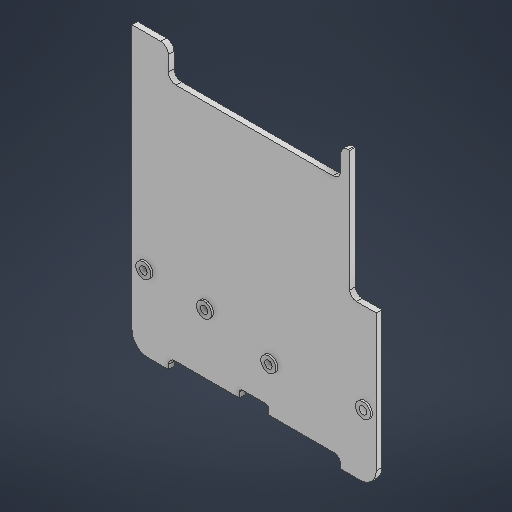
# Autodesk Inventor part: 第二层板
Saved by Autodesk Inventor 2025 (Build 290162000, 162)
## iProperties
Created: 2025-11-17
Part Number: 第二层板
Material: 常规
Document SubType Name: Modeling
Designer: XH
Density: 1 g/cm^3
Appearance: 默认
Author: XH
Autodesk Inventor part; units mm, degrees
ref_plane "YZ Plane" through (0, 0, 0) normal (1, 0, 0) x (0, 1, 0)
ref_plane "XZ Plane" through (0, 0, 0) normal (0, 1, 0) x (-1, 0, 0)
ref_plane "XY Plane" through (0, 0, 0) normal (0, 0, 1) x (1, 0, 0)
sketch "草图1" plane through (0, 0, 0) normal (0, 0, 1) x (1, 0, 0)
  arc A0 (28.0311, -36.5071) -> (33.0311, -31.5071) centre (28.0311, -31.5071) ccw
  line L0 (33.0311, -31.5071) -> (33.0311, 38.9929)
  line L1 (-32.9689, 38.9929) -> (-32.9689, -31.5071)
  arc A1 (-32.9689, -31.5071) -> (-27.9689, -36.5071) centre (-27.9689, -31.5071) ccw
  line L2 (3.8993, -36.5071) -> (3.8993, -31.5071)
  line L3 (3.8993, -36.5071) -> (28.0311, -36.5071)
  line L4 (-27.9689, -36.5071) -> (-3.837, -36.5071)
  line L5 (-3.837, -31.5071) -> (-3.837, -36.5071)
  spline S0 degree 3 poles (-2.9689, -30.724) (-3.0651, -30.724) (-3.1616, -30.7385) (-3.4015, -30.8136) (-3.5389, -30.8982) (-3.7629, -31.1465) (-3.837, -31.3265) (-3.837, -31.5071) knots 0 0 0 0 0.223691 0.223691 0.581598 0.581598 1 1 1 1
  line L6 (3.0311, -30.724) -> (-2.9689, -30.724)
  spline S1 degree 3 poles (3.8993, -31.5071) (3.8993, -31.3255) (3.8262, -31.1474) (3.5998, -30.8969) (3.4634, -30.8135) (3.224, -30.7385) (3.1274, -30.724) (3.0311, -30.724) knots 0 0 0 0 0.418614 0.418614 0.77639 0.77639 1 1 1 1
  line L7 (33.0311, 38.9929) -> (-32.9689, 38.9929)
  point P0 (22.1238, -37.5165)
extrude "拉伸1" add sketch "草图1" along normal blind 1.5
sketch "草图2" plane through (0, 0, 1.5) normal (0, 0, 1) x (1, 0, 0)
  line L0 (-21.8762, -36.6656) -> (22.1238, -36.6656)
  line L1 (22.1238, -36.6656) -> (-21.8762, -36.6656)
  line L2 (-21.8762, -36.6656) -> (-21.8762, -33.6656)
  line L3 (-21.8762, -33.6656) -> (22.1238, -33.6656)
  line L4 (22.1238, -33.6656) -> (22.1238, -36.6656)
  line L5 (-27.7974, -36.6656) -> (28.2026, -36.6656) projected
  point P0 (0, 0)
  point P1 (-21.8762, -36.6656)
  dimension "d3" = 3
  constraints: 10 end point, 2 parallel, 1 collinear, 1 horizontal, 1 perpendicular
  measures "d3" distance of L1.end L2.end
extrude "拉伸2" cut sketch "草图2" against normal blind 2
fillet "圆角1" radius 1 2 edges at (-21.8762, -33.6656, 0.75) (22.1238, -33.6656, 0.75)
sketch "草图3" plane through (0, 0, 1.5) normal (0, 0, 1) x (1, 0, 0)
  line L0 (26.0311, 37.3344) -> (33.1347, 37.3344)
  line L1 (33.0311, 37.4521) -> (33.0311, 5.3344)
  line L2 (33.0311, 5.3344) -> (26.0311, 5.3344)
  line L3 (26.0311, 5.3344) -> (26.0311, 37.3344)
  line L4 (33.0311, -31.5071) -> (33.0311, 38.9929) projected
  line L5 (33.2026, 37.3344) -> (-32.7974, 37.3344) projected
  point P0 (0, 0)
  point P1 (33.2026, -31.6656)
  point P2 (33.0311, 37.3344)
  point P3 (33.0311, 38.9929)
  dimension "d10" = 7
  dimension "d11" = 32
  constraints: 8 end point, 1 collinear, 1 horizontal, 1 parallel, 1 perpendicular, 1 vertical, 1 other
  measures "d10" distance between parallel lines of L1 L3
  measures "d11" distance between parallel lines of L0 L2
extrude "拉伸3" cut sketch "草图3" against normal blind 10
fillet "圆角2" radius 1 1 edges at (26.0311, 5.3344, 0.75)
sketch "草图4" plane through (0, 0, 1.5) normal (0, 0, 1) x (1, 0, 0)
  line L0 (33.0311, 5.3344) -> (27.0311, 5.3344) projected
  arc A0 (26.0311, 6.3344) -> (27.0311, 5.3344) centre (27.0311, 6.3344) ccw projected
  line L1 (26.0311, 6.3344) -> (26.0311, 37.3344) projected
  line L2 (-32.9689, 38.9929) -> (-32.9689, -31.5071) projected
  arc A1 (-32.9689, -31.5071) -> (-27.9689, -36.5071) centre (-27.9689, -31.5071) ccw projected
  line L3 (-21.8762, -36.5071) -> (-21.8762, -34.6656) projected
  arc A2 (-20.8762, -33.6656) -> (-21.8762, -34.6656) centre (-20.8762, -34.6656) ccw projected
  line L4 (-20.8762, -33.6656) -> (-3.837, -33.6656) projected
  arc A3 (22.1238, -34.6656) -> (21.1238, -33.6656) centre (21.1238, -34.6656) ccw projected
  line L5 (22.1238, -34.6656) -> (22.1238, -36.5071) projected
  arc A4 (28.0311, -36.5071) -> (33.0311, -31.5071) centre (28.0311, -31.5071) ccw projected
  line L6 (33.0311, -31.5071) -> (33.0311, 5.3344) projected
  line L7 (-32.2293, 38.2533) -> (25.2916, 38.2533)
  line L8 (25.2916, 38.2533) -> (25.2916, 6.3344)
  arc A5 (25.2916, 6.3344) -> (27.0311, 4.5949) centre (27.0311, 6.3344) ccw
  line L9 (27.0311, 4.5949) -> (32.2916, 4.5949)
  line L10 (32.2916, 4.5949) -> (32.2916, -31.5071)
  arc A6 (28.0311, -35.7676) -> (32.2916, -31.5071) centre (28.0311, -31.5071) ccw
  line L11 (28.0311, -35.7676) -> (22.8633, -35.7676)
  line L12 (22.8633, -35.7676) -> (22.8633, -34.6656)
  arc A7 (22.8633, -34.6656) -> (21.1238, -32.926) centre (21.1238, -34.6656) ccw
  line L13 (21.1238, -32.926) -> (-20.8762, -32.926)
  arc A8 (-20.8762, -32.926) -> (-22.6158, -34.6656) centre (-20.8762, -34.6656) ccw
  line L14 (-22.6158, -34.6656) -> (-22.6158, -35.7676)
  line L15 (-22.6158, -35.7676) -> (-27.9689, -35.7676)
  arc A9 (-32.2293, -31.5071) -> (-27.9689, -35.7676) centre (-27.9689, -31.5071) ccw
  line L16 (-32.2293, -31.5071) -> (-32.2293, 38.2533)
  line L17 (26.0311, 37.3344) -> (33.0311, 37.3344) projected
  line L18 (33.0311, 37.3344) -> (33.0311, 38.9929) projected
  line L19 (33.0311, 38.9929) -> (-32.9689, 38.9929) projected
  line L20 (-27.9689, -36.5071) -> (-21.8762, -36.5071) projected
  line L21 (-3.837, -33.6656) -> (-3.837, -31.5071) projected
  spline S0 degree 3 poles (-3.837, -31.5071) (-3.837, -31.3265) (-3.7629, -31.1465) (-3.5389, -30.8982) (-3.4015, -30.8136) (-3.1616, -30.7385) (-3.0651, -30.724) (-2.9689, -30.724) knots 0 0 0 0 0.418402 0.418402 0.776309 0.776309 1 1 1 1 projected
  line L22 (-2.9689, -30.724) -> (3.0311, -30.724) projected
  spline S1 degree 3 poles (3.0311, -30.724) (3.1274, -30.724) (3.224, -30.7385) (3.4634, -30.8135) (3.5998, -30.8969) (3.8262, -31.1474) (3.8993, -31.3255) (3.8993, -31.5071) knots 0 0 0 0 0.22361 0.22361 0.581386 0.581386 1 1 1 1 projected
  line L23 (3.8993, -31.5071) -> (3.8993, -33.6656) projected
  line L24 (3.8993, -33.6656) -> (21.1238, -33.6656) projected
  line L25 (22.1238, -36.5071) -> (28.0311, -36.5071) projected
  point P0 (0, 0)
  constraints: 20 end point, 10 point on circle, 5 centre point, 11 other
extrude "拉伸4" cut sketch "草图4" against normal blind 10 contours L6 A4 L25 L5 A3 L24 L23 L13 A7 L12 L11 A6 L10 L9 A5 L8 L7 L16 A9 L15 L14 A8 L21 L4 A2 L3 L20 A1 L2 L19 L18 L17 L1 A0 L0
sketch "草图5" plane through (0, 0, 1.5) normal (0, 0, 1) x (1, 0, 0)
  line L0 (25.2916, 38.2533) -> (-32.2293, 38.2533) projected
  line L1 (-22.6158, -35.7676) -> (22.8633, -35.7676)
  line L2 (22.8633, -35.7676) -> (22.8633, 38.2533)
  line L3 (22.8633, 38.2533) -> (-22.6158, 38.2533)
  line L4 (-22.6158, 38.2533) -> (-22.6158, -35.7676)
  line L5 (22.8633, -34.6656) -> (22.8633, -35.7676) projected
  line L6 (-22.6158, -35.7676) -> (-22.6158, -34.6656) projected
  line L7 (-27.9689, -35.7676) -> (-22.6158, -35.7676) projected
  line L8 (-22.6158, 30.2533) -> (22.8633, 30.2533)
  point P0 (0, 0)
  point P1 (-22.6158, 38.2533)
  dimension "d16" = 8
  constraints: 10 end point, 3 collinear, 3 point on line, 2 parallel, 2 perpendicular, 1 horizontal
  measures "d16" distance between parallel lines of L3 L8
extrude "拉伸5" cut sketch "草图5" against normal blind 10 contours L2 L8 L4 L0
fillet "圆角3" radius 2 4 edges at (22.8633, 38.2533, 0.75) (22.8633, 30.2533, 0.75) (-22.6158, 38.2533, 0.75) (-22.6158, 30.2533, 0.75)
sketch "草图6" plane through (0, 0, 1.5) normal (0, 0, 1) x (1, 0, 0)
  line L0 (29.89, -22.1052) -> (29.89, -32.1052) projected
  line L1 (29.89, -32.1052) -> (18.89, -32.1052) projected
  line L2 (18.89, -32.1052) -> (18.89, -22.1052) projected
  line L3 (18.89, -22.1052) -> (29.89, -22.1052) projected
  circle A0 centre (-28.7084, -15.9176) radius 1
  circle A1 centre (29.2916, -18.9176) radius 1
  circle A2 centre (-12.7084, -16.9176) radius 1
  circle A3 centre (4.2916, -20.9176) radius 1
  line L4 (-32.11, -33.9176) -> (31.89, -33.9176) projected
  line L5 (31.89, -33.9176) -> (31.89, 6.0824) projected
  line L6 (31.89, 6.0824) -> (-32.11, 6.0824) projected
  line L7 (-32.11, 6.0824) -> (-32.11, -33.9176) projected
  circle A4 centre (-28.7084, -15.9176) radius 2
  circle A5 centre (-12.7084, -16.9176) radius 2
  circle A6 centre (4.2916, -20.9176) radius 2
  circle A7 centre (29.2916, -18.9176) radius 2
  line L8 (-27.9689, -35.7676) -> (-22.6158, -35.7676) projected
  line L9 (-20.8762, -32.926) -> (-3.837, -32.926) projected
  line L10 (3.8993, -32.926) -> (21.1238, -32.926) projected
  line L11 (22.8633, -35.7676) -> (28.0311, -35.7676) projected
  line L12 (32.2916, -31.5071) -> (32.2916, 4.5949) projected
  point P0 (0, 0)
  point P1 (-25.2923, -35.7676)
  point P2 (-12.3566, -32.926)
  dimension "d20" = 1
  dimension "d21" = 1
  dimension "d22" = 1
  dimension "d23" = 1
  dimension "d28" = 25
  dimension "d29" = 17
  dimension "d30" = 16
  dimension "d31" = 19.8499
  dimension "d32" = 16.0084
  dimension "d33" = 12.0084
  dimension "d34" = 16.8499
  dimension "d35" = 3
  constraints: 8 centre point, 2 midpoint
  measures "d20" radial gap between concentric circles of A0 A4
  measures "d21" radial gap between concentric circles of A2 A5
  measures "d22" radial gap between concentric circles of A3 A6
  measures "d23" radial gap between concentric circles of A1 A7
  measures "d28" horizontal distance of A3.centre A1.centre
  measures "d29" horizontal distance of A3.centre A2.centre
  measures "d30" horizontal distance of A2.centre A0.centre
  measures "d31" vertical distance of point (-25.292, -35.768) A0.centre
  measures "d32" vertical distance of point (-12.357, -32.926) A2.centre
  measures "d33" distance from line of L10 A3.centre
  measures "d34" distance from line of L11 A1.centre
  measures "d35" distance from line of A1.centre L12
extrude "拉伸7" add sketch "草图6" along normal blind 0.5 contours A4 | A5 | A6 | A7
sketch "草图7" plane through (-28.7084, -15.9176, 1.5) normal (0, 0, 1) x (1, 0, 0)
  circle A0 centre (16, -1) radius 1 projected
  circle A1 centre (0, 0) radius 1 projected
  circle A2 centre (33, -5) radius 1 projected
  circle A3 centre (58, -3) radius 1 projected
  point P0 (28.7084, 15.9176)
extrude "拉伸8" cut sketch "草图7" against normal blind 7
